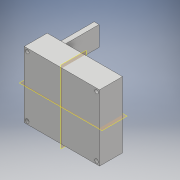
# Autodesk Inventor part: board
Saved by Autodesk Inventor 2019 (Build 230136000, 136)
## iProperties
Created: 2018-07-19
Part Number: board
Material: Générique
Document SubType Name: Modeling
Designer: julien.allali
Density: 1 g/cm^3
Appearance: Par défaut
Author: julien.allali
Autodesk Inventor part; units mm, degrees
ref_plane "YZ Plane" through (0, 0, 0) normal (1, 0, 0) x (0, 1, 0)
ref_plane "XZ Plane" through (0, 0, 0) normal (0, 1, 0) x (-1, 0, 0)
ref_plane "XY Plane" through (0, 0, 0) normal (0, 0, 1) x (1, 0, 0)
sketch "Sketch1" plane through (0, 0, 0) normal (0, 1, 0) x (-1, 0, 0)
  line L0 (0, 0) -> (62.35, 0)
  line L1 (62.35, 0) -> (62.35, -54.68)
  line L2 (62.35, -54.68) -> (0, -54.68)
  line L3 (0, -54.68) -> (0, 0)
  dimension "d0" = 54.68
  dimension "d1" = 62.35
  constraints: 8 end point, 2 parallel, 1 horizontal, 1 perpendicular
  measures "d0" distance of L0.end L1.end
  measures "d1" distance of L1.end L2.end
extrude "Extrusion1" add sketch "Sketch1" along normal blind 19
sketch "Sketch2" plane through (0, 19, 0) normal (0, 1, 0) x (1, 0, 0)
  line L0 (-62.35, 54.68) -> (-62.35, 0) projected
  line L1 (0, 54.68) -> (-62.35, 54.68) projected
  point P0 (0, 0)
  point P1 (-59.85, 52.18)
  dimension "d4" = 2.5
  dimension "d5" = 2.5
  measures "d4" distance from line of L0 point (-59.85, 52.18)
  measures "d5" distance from line of L1 point (-59.85, 52.18)
hole "Hole1" at (-59.85, 19, -52.18) direction (0, -1, 0) diameter 3 end through all
ref_plane "Work Plane1" through (-62.35, 0, -27.34) normal (0, 0, 1) x (1, 0, 0)
ref_plane "Work Plane2" through (-31.175, 0, 0) normal (1, 0, 0) x (0, 0, -1)
mirror "Mirror1" about plane through (-62.35, 0, -27.34) normal (0, 0, 1) of "Hole1"
mirror "Mirror2" about plane through (-31.175, 0, 0) normal (1, 0, 0) of "Hole1", "Mirror1"
sketch "Sketch3" plane through (0, 19, 0) normal (0, 1, 0) x (1, 0, 0)
  line L0 (-48.05, 1) -> (-52.05, 1)
  line L1 (-52.05, 1) -> (-52.05, 17.4)
  line L2 (-52.05, 17.4) -> (-48.05, 17.4)
  line L3 (-48.05, 17.4) -> (-48.05, 1)
  line L4 (-62.35, 0) -> (0, 0) projected
  line L5 (-62.35, 54.68) -> (-62.35, 0) projected
  dimension "d13" = 4
  dimension "d14" = 16.4
  dimension "d15" = 1
  dimension "d16" = 10.3
  constraints: 8 end point, 2 parallel, 1 horizontal, 1 perpendicular
  measures "d13" distance of L0.start L0.end
  measures "d14" distance of L0.end L1.end
  measures "d15" distance between parallel lines of L4 L0
  measures "d16" distance between parallel lines of L5 L1
extrude "Extrusion2" add sketch "Sketch3" along normal blind 28.6
sketch "Sketch4" plane through (0, 19, 0) normal (0, 1, 0) x (1, 0, 0)
  circle A0 centre (-5.7, 9) radius 2.75
  line L0 (-62.35, 0) -> (0, 0) projected
  line L1 (0, 0) -> (0, 54.68) projected
  dimension "d19" = 5.5
  dimension "d20" = 9
  dimension "d21" = 5.7
  constraints: 1 centre point
  measures "d19" diameter of A0
  measures "d20" distance from line of A0.centre L0
  measures "d21" distance from line of L1 A0.centre
extrude "Extrusion3" cut sketch "Sketch4" against normal blind 10
equation "\"d5\" = d4"
body "Solid1"
